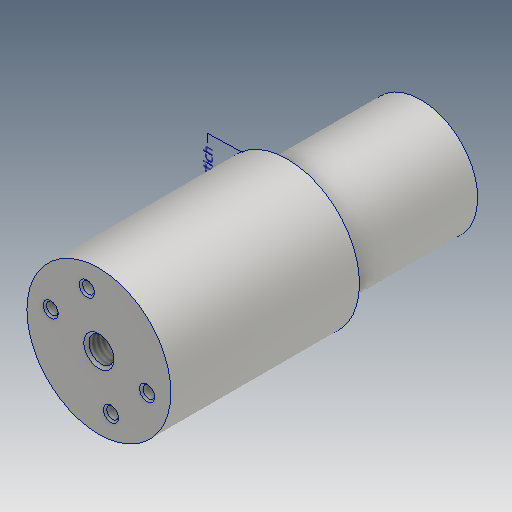
# Autodesk Inventor part: 200-20-ROCKER-CONNECTOR-01
Saved by Autodesk Inventor 2018.2 (Build 222227000, 227)
## iProperties
Manager: feesmrt
Company: FRANC0R
Created: 2017-10-30
Part Number: 200-20-ROCKER-CONNECTOR-01
Material: Aluminium 6061
Document SubType Name: Modeling
Designer: feesmrt
Density: 2.7 g/cm^3
Appearance: Aluminium - flach
Project: Rescue Robot
Cost Center: -
Description: Rocker Profile Connector
Engineer: feesmrt
Authority: feesmrt
Stock Number: 200-20-ROCKER-CONNECTOR-01
Author: feesmrt
Title: Rocker Profile Connector
Subject: Rescue Robot
Revision Number: 1
Autodesk Inventor part; units mm, degrees
ref_plane "YZ Plane" through (0, 0, 0) normal (1, 0, 0) x (0, 1, 0)
ref_plane "XZ Plane" through (0, 0, 0) normal (0, 1, 0) x (-1, 0, 0)
ref_plane "XY Plane" through (0, 0, 0) normal (0, 0, 1) x (1, 0, 0)
derived "200-10-ROCKER-BEARING-01.ipt"
sketch "Skizze_Lagersitz" plane through (0, 0, 0) normal (1, 0, 0) x (0, 1, 0)
  line L0 (-12.5, 36) -> (32.5, 36)
  line L1 (-12.5, -36) -> (-12.5, 36)
  line L2 (-17.5, 32.25) -> (-12.5, 32.25)
  line L3 (-17.5, -32.25) -> (-17.5, 32.25)
  line L4 (-32.5, 18) -> (-17.5, 18)
  line L5 (-32.5, -18) -> (-17.5, -18)
  line L6 (-17.5, -32.25) -> (-12.5, -32.25)
  line L7 (-12.5, -36) -> (32.5, -36)
  line L8 (32.5, 36) -> (32.5, -36)
  line L9 (32.5, 50) -> (32.5, -50)
  line L10 (30, -50) -> (30, 0)
  line L11 (-32.5, -18) -> (-32.5, 18)
  line L12 (-32.5, 50) -> (-32.5, -50)
  line L13 (-32.5, -50) -> (-32.5, 50)
  line L14 (-12.5, -36) -> (-12.5, 36)
  point P0 (0, 0)
  point P1 (30, 86)
  point P2 (30, 14)
  point P3 (-30, 32)
  point P4 (-30, 68)
sketch "Skizze4" plane through (0, 0, 0) normal (1, 0, 0) x (0, 1, 0)
  line L0 (-81.26, 0) -> (51.46, 0) projected
  line L1 (-12.5, -36) -> (-12.5, 36) construction
  line L2 (-32.5, -18) -> (-32.5, 18) construction
  line L3 (22.7, 0) -> (22.7, 15)
  line L4 (22.7, 15) -> (-12.5, 15)
  line L5 (17.7, 0) -> (17.7, 36) construction
  line L6 (-12.5, 15) -> (-12.5, 19)
  line L7 (-12.5, 19) -> (-62.3, 19)
  line L8 (-62.3, 0) -> (22.7, 0)
  line L9 (-62.3, 19) -> (-62.3, 0)
  line L10 (-12.5, 36) -> (32.5, 36) construction
  point P0 (0, 0)
  dimension "d3" = 30.2
  dimension "d4" = 5
  dimension "d5" = 30
  dimension "d6" = 38
  dimension "d7" = 85
  constraints: 14 end point, 6 point on line, 2 horizontal, 2 vertical, 1 collinear, 1 perpendicular
  measures "d3" distance between parallel lines of L5 L1
  measures "d4" distance between parallel lines of L3 L5
  measures "d5" diameter of L4 L0
  measures "d6" diameter of L7 L0
  measures "d7" distance from line of L7.end L3
revolve "Grundkoerper" add sketch "Skizze4" angle 360 about axis through (0, 0, 0) along (0, 1, 0)
sketch "Skizze11" plane through (0, -62.3, 0) normal (0, -1, 0) x (1, 0, 0)
  circle A0 centre (0, 0) radius 19 projected
hole "M6x12_CubeConn" at (0, -62.3, 0) direction (0, 1, 0) diameter 6.647 depth 22.2 tip angle 118 countersink diameter 8 countersink angle 90 thread size "M8x1.25" class "6H" standard "ISO Metric profile"
sketch "Skizze13" plane through (0, -62.3, 0) normal (0, -1, 0) x (1, 0, 0)
  line L0 (0, 113.2) -> (0, -77.2) construction
  line L1 (-26.6, 0) -> (26.6, 0) construction
  circle A0 centre (0, 0) radius 3
  line L2 (12.7279, -3.182) -> (-3.182, 12.7279) construction
  line L3 (-3.182, 12.7279) -> (-12.7279, 3.182) construction
  line L4 (-12.7279, 3.182) -> (3.182, -12.7279) construction
  line L5 (3.182, -12.7279) -> (12.7279, -3.182) construction
  line L6 (12.7279, -3.182) -> (-12.7279, 3.182) construction
  line L7 (-3.182, 12.7279) -> (3.182, -12.7279) construction
  line L8 (7.955, -7.955) -> (-7.955, 7.955) construction
  point P0 (0, 0)
  point P1 (-3.182, 12.7279)
  point P2 (12.7279, -3.182)
  point P3 (3.182, -12.7279)
  dimension "d98" = 22.5
  dimension "d99" = 13.5
  dimension "d100" = 6
  dimension "d102" = 45
  constraints: 14 end point, 5 midpoint, 4 coincident, 2 parallel, 1 centre point, 1 perpendicular
  measures "d98" distance of L2.start L2.end
  measures "d99" distance of L2.end L3.end
  measures "d100" diameter of A0
  measures "d102" angle of L0 L8
hole "Hole_3,1x6" at (-12.7279, -62.3, 3.182) at (-3.182, -62.3, 12.7279) at (12.7279, -62.3, -3.182) at (3.182, -62.3, -12.7279) direction (0, 1, 0) diameter 3.1 depth 8 tip angle 118 countersink diameter 4 countersink angle 90
sketch "Skizze14" plane through (0, 22.7, 0) normal (0, 1, 0) x (1, 0, 0)
  circle A0 centre (0, 0) radius 15 construction
  constraints: 1 coincident
hole "M6x12_BearingFix" at (0, 22.7, 0) direction (0, -1, 0) diameter 4.917 depth 17.1 tip angle 118 countersink diameter 6 countersink angle 90 thread size "M6x1" class "6H" standard "ISO Metric profile"
